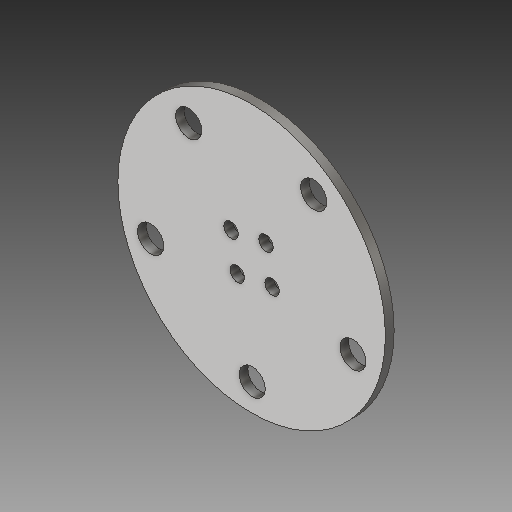
# Autodesk Inventor part: WheelHub
Saved by Autodesk Inventor 2017 (Build 210142000, 142)
## iProperties
Created: 2017-02-04
Part Number: WheelHub
Material: Steel, Mild
Document SubType Name: Sheet Metal
Designer: Robert.Chapman
Density: 7.85 g/cm^3
Sheet Metal Rule: Default
Appearance: Semi-Polished
Author: Robert.Chapman
Autodesk Inventor part; units mm, degrees
ref_plane "YZ Plane" through (0, 0, 0) normal (1, 0, 0) x (0, 1, 0)
ref_plane "XZ Plane" through (0, 0, 0) normal (0, 1, 0) x (-1, 0, 0)
ref_plane "XY Plane" through (0, 0, 0) normal (0, 0, 1) x (1, 0, 0)
sketch "Sketch1" plane through (0, 0, 0) normal (0, 0, 1) x (1, 0, 0)
  circle A0 centre (0, 0) radius 73.025
  dimension "d7" = 146.05
  measures "d7" diameter of A0
extrude "Plate1" add sketch "Sketch1" along normal blind 4.7625
sketch "Sketch2" plane through (0, 0, 4.7625) normal (0, 0, 1) x (1, 0, 0)
  circle A0 centre (-11.2011, 7.8489) radius 3.9688
  circle A1 centre (-7.8489, -11.2011) radius 3.9688
  circle A2 centre (11.2011, -7.8489) radius 3.9688
  circle A3 centre (7.8489, 11.2011) radius 3.9688
  point P0 (0, 0)
  dimension "d8" = 7.9375
  dimension "d11" = 360
  dimension "d20" = 19.05
  constraints: 4 centre point, 9 other
  measures "d8" diameter of A0
  measures "d20" horizontal distance of A3.centre A0.centre
hole "Hole1" at (-11.2011, 7.8489, 4.7625) at (7.8489, 11.2011, 4.7625) at (-7.8489, -11.2011, 4.7625) at (11.2011, -7.8489, 4.7625) direction (0, 0, -1) diameter 7.9375 end through all
sketch "Sketch3" plane through (0, 0, 4.7625) normal (0, 0, 1) x (1, 0, 0)
  circle A0 centre (-34.3723, 46.8025) radius 6.498 construction
  circle A1 centre (-55.1334, -18.2273) radius 6.498 construction
  circle A2 centre (0.298, -58.0676) radius 6.498 construction
  circle A3 centre (55.3176, -17.6604) radius 6.498 construction
  circle A4 centre (33.8902, 47.1528) radius 6.498 construction
  point P0 (0, 0)
  dimension "d21" = 12.9959
  dimension "d24" = 360
  dimension "d33" = 68.2625
  constraints: 5 centre point, 11 other
  measures "d21" diameter of A0
  measures "d33" horizontal distance of A4.centre A0.centre
hole "Hole2" at (33.8902, 47.1528, 4.7625) at (55.3176, -17.6604, 4.7625) at (0.298, -58.0676, 4.7625) at (-55.1334, -18.2273, 4.7625) at (-34.3723, 46.8025, 4.7625) direction (0, 0, -1) diameter 14.2875 end through all
equation "\"d18\" = Thickness"
equation "\"d31\" = Thickness"
equation "\"BendRadius\" = Thickness"
equation "\"BendReliefWidth\" = Thickness"
equation "\"BendReliefDepth\" = 0.5 * Thickness"
equation "\"CornerReliefSize\" = 4 * Thickness"
equation "\"MinimumRemnant\" = 2 * Thickness"
equation "\"TransitionRadius\" = BendRadius"
equation "\"JacobiRadiusSize\" = BendRadius"
equation "\"GapSize\" = Thickness"
equation "\"d0\" = BendRadius"
equation "\"Thickness\" = 4.7625"
body "Solid1"
